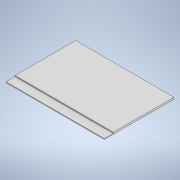
# Autodesk Inventor part: False_Bottom_4
Saved by Autodesk Inventor 2020 (Build 240168000, 168)
## iProperties
Created: 2022-01-22
Part Number: False_Bottom_4
Material: Generic
Document SubType Name: Modeling
Designer: danie
Density: 1 g/cm^3
Appearance: Default
Author: danie
Autodesk Inventor part; units mm, degrees
ref_plane "YZ Plane" through (0, 0, 0) normal (1, 0, 0) x (0, 1, 0)
ref_plane "XZ Plane" through (0, 0, 0) normal (0, 1, 0) x (-1, 0, 0)
ref_plane "XY Plane" through (0, 0, 0) normal (0, 0, 1) x (1, 0, 0)
sketch "Sketch1" plane through (0, 0, 0) normal (0, 1, 0) x (-1, 0, 0)
  line L0 (0, 0) -> (0, -86.36)
  line L1 (0, -86.36) -> (-139.7, -86.36)
  line L2 (-139.7, -86.36) -> (-139.7, 0)
  line L3 (-139.7, 0) -> (0, 0)
  line L4 (0, 0) -> (86.36, 0) construction
  dimension "d0" = 86.36
  dimension "d1" = 90
  dimension "d2" = 139.7
  constraints: 10 end point, 2 parallel, 2 perpendicular, 1 horizontal, 1 vertical
  measures "d0" distance of L0.start L0.end
  measures "d1" angle of L0 L4
  measures "d2" distance of L0.end L1.end
extrude "Extrusion1" add sketch "Sketch1" along normal blind 2.54
sketch "Sketch2" plane through (0, 0, 0) normal (0, 0, 1) x (1, 0, 0)
  line L0 (0, 0) -> (139.7, 0) projected
  line L1 (0, 0) -> (139.7, 0)
  line L2 (139.7, 0) -> (139.7, 1.27)
  line L3 (139.7, 1.27) -> (0, 1.27)
  line L4 (0, 1.27) -> (0, 0)
  dimension "d5" = 1.27
  constraints: 8 end point, 3 equal length, 1 perpendicular
  measures "d5" distance of L2.end L0.end
extrude "Extrusion2" add sketch "Sketch2" along normal blind 12.7
body "Solid1"
